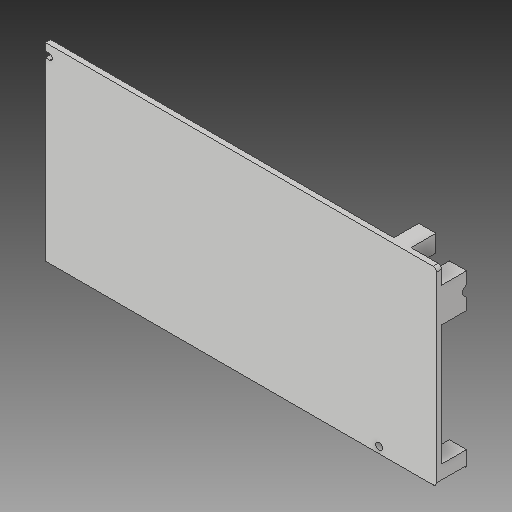
# Autodesk Inventor part: PowerS_case
Saved by Autodesk Inventor 2019.3 (Build 233278000, 278)
## iProperties
Created: 2020-08-31
Part Number: PowerS_case
Material: Generisch
Document SubType Name: Modeling
Designer: Nicolas Frick
Density: 1 g/cm^3
Appearance: Vorgabe
Author: Nicolas Frick
Autodesk Inventor part; units mm, degrees
ref_plane "YZ Plane" through (0, 0, 0) normal (1, 0, 0) x (0, 1, 0)
ref_plane "XZ Plane" through (0, 0, 0) normal (0, 1, 0) x (-1, 0, 0)
ref_plane "XY Plane" through (0, 0, 0) normal (0, 0, 1) x (1, 0, 0)
sketch "Skizze1" plane through (0, 0, 0) normal (0, 0, 1) x (1, 0, 0)
  line L0 (-99.499, 50.6459) -> (-97.0783, 50.6459) projected
  arc A0 (-97.0783, 47.3459) -> (-97.0783, 50.6459) centre (-97.0783, 48.9959) ccw projected
  line L1 (-97.0783, 47.3459) -> (-99.499, 47.3459) projected
  line L2 (-99.499, 47.3459) -> (-99.499, -55.0406) projected
  line L3 (-99.499, -55.0406) -> (-92.499, -55.0406) projected
  line L4 (-92.499, -55.0406) -> (-92.499, -54.9737) projected
  line L5 (-92.499, -54.9737) -> (83.501, -54.9737) projected
  line L6 (83.501, -54.9737) -> (83.501, -55.0406) projected
  line L7 (83.501, -55.0406) -> (99.501, -55.0406) projected
  line L8 (99.501, 55.0263) -> (-99.499, 55.0263) projected
  line L9 (-99.499, 55.0263) -> (-99.499, 50.6459) projected
  circle A1 centre (94.5371, -51.3279) radius 2 projected
  circle A2 centre (39.415, 44.5055) radius 1.5 construction
  circle A3 centre (-86.3913, -41.8325) radius 1.5 construction
  circle A4 centre (39.415, -41.8325) radius 1.5 construction
  circle A5 centre (-86.3913, 44.5055) radius 1.5 construction
  line L10 (99.501, 55.0263) -> (127.8857, 55.0263)
  line L11 (127.8857, 55.0263) -> (127.8857, -55.0406)
  line L12 (127.8857, -55.0406) -> (99.501, -55.0406)
  line L13 (99.501, -55.0406) -> (99.501, 55.0263) construction
  line L14 (127.8857, 55.0263) -> (-99.499, 55.0263)
  line L15 (-99.499, 55.0263) -> (-99.499, -55.0406)
  line L16 (-99.499, -55.0406) -> (127.8857, -55.0406)
  line L17 (127.8857, -55.0406) -> (127.8857, 55.0263)
  point P0 (0, 0)
  constraints: 16 end point, 4 parallel, 2 horizontal, 2 perpendicular
extrude "Extrusion1" add sketch "Skizze1" along normal blind 3 contours L9 L8 L10 L11 L12 L7 L6 L5 L4 L3 L2 L1 A0 L0 | L4 L5 L6 L16
sketch "Skizze2" plane through (0, 0, 0) normal (0, 0, -1) x (-1, 0, 0)
  line L0 (-84.9297, 45.0263) -> (-99.501, 45.0263) construction
  line L1 (-99.501, 45.0263) -> (-99.501, -44.3215) construction
  line L2 (-99.501, -44.3215) -> (-84.9297, -44.3215) construction
  line L3 (-84.9297, -44.3215) -> (-84.9297, 45.0263) construction
  line L4 (-127.8857, -55.0406) -> (-127.8857, 55.0263) construction
  line L5 (-127.8857, 45.0263) -> (-117.8857, 45.0263)
  line L6 (-117.8857, 45.0263) -> (-117.8857, 25.0263)
  line L7 (-117.8857, 25.0263) -> (-127.8857, 25.0263)
  line L8 (-127.8857, 25.0263) -> (-127.8857, 45.0263)
  point P0 (0, 0)
  dimension "d2" = 10
  dimension "d3" = 20
  constraints: 8 end point, 2 parallel, 1 horizontal, 1 perpendicular, 1 point on line
  measures "d2" distance of L6.end L7.end
  measures "d3" distance of L5.end L6.end
extrude "Extrusion2" add sketch "Skizze2" along normal blind 14.5
sketch "Skizze3" plane through (127.8857, -55.0406, 3) normal (1, 0, 0) x (0, 0, -1)
  line L0 (17.5, 100.0669) -> (17.5, 80.0669) projected
  arc A0 (17.5, 92.5669) -> (17.5, 87.5669) centre (17.5, 90.0669) ccw
  line L1 (17.5, 92.5669) -> (17.5, 87.5669)
  point P0 (3, 55.0406)
  dimension "d6" = 5
  constraints: 2 end point, 2 point on circle, 2 point on line, 1 centre point, 1 midpoint
  measures "d6" diameter of A0
extrude "Extrusion3" cut sketch "Skizze3" against normal blind 14.5
fillet "Rundung1" radius 2 2 edges at (122.8857, 32.5263, -14.5) (122.8857, 37.5263, -14.5)
sketch "Skizze4" plane through (0, 0, -14.5) normal (0, 0, -1) x (-1, 0, 0)
  line L0 (-117.8857, 39.0574) -> (-127.8857, 39.0574) projected
  line L1 (-117.8857, 39.0574) -> (-117.8857, 45.0263) projected
  line L2 (-117.8857, 45.0263) -> (-127.8857, 45.0263) projected
  line L3 (-127.8857, 45.0263) -> (-127.8857, 39.0574) projected
  line L4 (-127.8857, 30.9952) -> (-117.8857, 30.9952) projected
  line L5 (-127.8857, 30.9952) -> (-127.8857, 25.0263) projected
  line L6 (-127.8857, 25.0263) -> (-117.8857, 25.0263) projected
  line L7 (-117.8857, 25.0263) -> (-117.8857, 30.9952) projected
  point P0 (0, 0)
  point P1 (-122.8857, 28.0107)
  point P2 (-122.8857, 42.0419)
hole "Bohrung1" at (122.8857, 28.0107, -14.5) at (122.8857, 42.0419, -14.5) direction (0, 0, 1) diameter 2.5 depth 10
sketch "Skizze6" plane through (0, 0, -14.5) normal (0, 0, -1) x (-1, 0, 0)
  line L0 (-127.8857, 37.2658) -> (-117.8857, 37.2658) projected
  line L1 (-127.8857, 32.7868) -> (-127.8857, 37.2658) projected
  line L2 (-117.8857, 32.7868) -> (-127.8857, 32.7868) projected
  line L3 (-117.8857, 37.2658) -> (-117.8857, 32.7868) projected
  line L4 (-127.8857, -55.0406) -> (-127.8857, 55.0263) projected
  line L5 (-127.8857, 35.0263) -> (-117.8857, 35.0263) construction
  line L6 (-127.8857, 35.3004) -> (-117.8857, 35.3004)
  line L7 (-117.8857, 35.3004) -> (-117.8857, 34.7646)
  line L8 (-117.8857, 34.7646) -> (-127.8857, 34.7646)
  line L9 (-127.8857, 34.7646) -> (-127.8857, 35.3004)
  point P0 (0, 0)
  constraints: 10 end point, 3 point on line, 2 parallel, 1 horizontal, 1 midpoint, 1 perpendicular
extrude "Extrusion4" add sketch "Skizze6" against normal up to surface contours L6 L3 L8 L1 round surface about axis through (127.8857, 35.0263, -14.5) along (-1, 0, 0) radius 2.5 far side no
sketch "Skizze7" plane through (127.8857, -55.0406, 3) normal (1, 0, 0) x (0, 0, -1)
  line L0 (17.5, 90.341) -> (15.0151, 90.341) projected
  line L1 (17.5, 89.8052) -> (15.0137, 89.8052) projected
  line L2 (17.5, 90.341) -> (15.3337, 90.341)
  line L3 (15.3337, 90.341) -> (15.3337, 89.8052)
  line L4 (15.3337, 89.8052) -> (17.5, 89.8052)
  line L5 (17.5, 89.8052) -> (17.5, 90.341)
  point P0 (3, 55.0406)
  constraints: 8 end point, 2 parallel, 1 horizontal, 1 perpendicular, 1 point on line
extrude "Extrusion5" cut sketch "Skizze7" against normal up to next
fillet "Rundung2" radius 2 2 edges at (127.8857, -55.0406, 1.5) (127.8857, 55.0263, 1.5)
sketch "Skizze8" plane through (0, 0, 0) normal (0, 0, -1) x (-1, 0, 0)
  line L0 (92.499, 55.0263) -> (-83.501, 55.0263) construction
  line L1 (-83.501, 55.0263) -> (-83.501, -54.9737) construction
  line L2 (-83.501, -54.9737) -> (-99.501, -54.9737) construction
  line L3 (-99.501, -54.9737) -> (-99.501, -56.2737) construction
  line L4 (99.5199, -56.2737) -> (-99.501, -56.2737) construction
  line L5 (99.5199, -54.9737) -> (99.5199, -56.2737) construction
  line L6 (99.5199, -54.9737) -> (92.499, -54.9737) construction
  line L7 (92.499, -54.9737) -> (92.499, 55.0263) construction
  line L8 (-84.9297, 45.0263) -> (-99.501, 45.0263) construction
  line L9 (-99.501, 45.0263) -> (-99.501, -44.3215) construction
  line L10 (-99.501, -44.3215) -> (-84.9297, -44.3215) construction
  line L11 (-84.9297, -44.3215) -> (-84.9297, 45.0263) construction
  line L12 (-127.8857, -55.0406) -> (-117.8857, -55.0406)
  line L13 (-117.8857, -55.0406) -> (-117.8857, -45.0406)
  line L14 (-117.8857, -45.0406) -> (-127.8857, -45.0406)
  line L15 (-127.8857, -45.0406) -> (-127.8857, -55.0406)
  line L16 (-99.501, 55.0263) -> (-99.501, 45.0263) construction
  line L17 (-99.501, -44.3215) -> (-99.501, -54.9737) construction
  line L18 (-125.8857, 55.0263) -> (99.499, 55.0263) projected
  line L19 (-110.0873, 55.0263) -> (-100.0873, 55.0263)
  line L20 (-100.0873, 55.0263) -> (-100.0873, 45.0263)
  line L21 (-100.0873, 45.0263) -> (-110.0873, 45.0263)
  line L22 (-110.0873, 45.0263) -> (-110.0873, 55.0263)
  point P0 (0, 0)
  dimension "d23" = 10
  dimension "d24" = 10
  dimension "d25" = 10
  constraints: 16 end point, 4 parallel, 2 horizontal, 2 perpendicular, 1 point on line
  measures "d23" distance of L14.end L13.end
  measures "d24" distance of L13.end L12.end
  measures "d25" distance of L20.end L21.end
extrude "Extrusion6" add sketch "Skizze8" along normal blind 14.5
fillet "Rundung3" radius 2 1 edges at (127.8857, -55.0406, -7.25)
sketch "Skizze9" plane through (0, 0, -14.5) normal (0, 0, -1) x (-1, 0, 0)
  line L0 (-100.0873, 55.0263) -> (-110.0873, 55.0263) projected
  line L1 (-110.0873, 55.0263) -> (-110.0873, 45.0263) projected
  line L2 (-110.0873, 45.0263) -> (-100.0873, 45.0263) projected
  line L3 (-100.0873, 45.0263) -> (-100.0873, 55.0263) projected
  arc A0 (-127.8857, -53.0406) -> (-125.8857, -55.0406) centre (-125.8857, -53.0406) ccw projected
  line L4 (-125.8857, -55.0406) -> (-117.8857, -55.0406) projected
  line L5 (-117.8857, -55.0406) -> (-117.8857, -45.0406) projected
  line L6 (-117.8857, -45.0406) -> (-127.8857, -45.0406) projected
  line L7 (-127.8857, -45.0406) -> (-127.8857, -53.0406) projected
  circle A1 centre (-105.0873, 50.0263) radius 1.75
  circle A2 centre (-122.8857, -50.0406) radius 1.75
  point P0 (0, 0)
  dimension "d29" = 3.5
  dimension "d30" = 3.5
  constraints: 2 centre point
  measures "d29" diameter of A1
  measures "d30" diameter of A2
extrude "Extrusion7" cut sketch "Skizze9" against normal blind 10 contours A1 | A2
